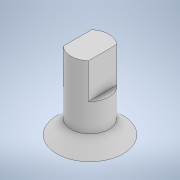
# Autodesk Inventor part: driven gear axle
Saved by Autodesk Inventor 2022 (Build 260153000, 153)
## iProperties
Created: 2021-11-11
Part Number: driven gear axle
Material: Generic
Document SubType Name: Modeling
Designer: a-dubs
Density: 1 g/cm^3
Appearance: Default
Author: a-dubs
Autodesk Inventor part; units mm, degrees
ref_plane "YZ Plane" through (0, 0, 0) normal (1, 0, 0) x (0, 1, 0)
ref_plane "XZ Plane" through (0, 0, 0) normal (0, 1, 0) x (-1, 0, 0)
ref_plane "XY Plane" through (0, 0, 0) normal (0, 0, 1) x (1, 0, 0)
sketch "Sketch1" plane through (0, 0, 0) normal (0, 1, 0) x (-1, 0, 0)
  line L0 (0, 0) -> (1.8, 0)
  line L1 (0, 0) -> (-1.8, 0)
  circle A0 centre (0, 0) radius 2.7
  line L2 (1.8, 0) -> (1.8, 2.0125)
  line L3 (1.8, 0) -> (1.8, -2.0125)
  line L4 (-1.8, 0) -> (-1.8, -2.0125)
  line L5 (-1.8, 0) -> (-1.8, 2.0125)
  circle A1 centre (0, 0) radius 4.7
  dimension "d0" = 1.8
  dimension "d1" = 1.8
  dimension "d2" = 5.4
  dimension "d7" = 9.4
  constraints: 12 end point, 4 point on circle, 2 centre point, 2 coincident, 2 horizontal, 2 point on line, 1 parallel, 1 vertical
  measures "d0" distance of L0.start L0.end
  measures "d1" distance of L0.start L1.end
  measures "d2" diameter of A0
  measures "d7" diameter of A1
extrude "Extrusion1" add sketch "Sketch1" along normal blind 4 contours L1 L5 A0 L2 L0 | L0 L3 A0 L4 L1 | L2 A0 L3 | L4 A0 L5
extrude "Extrusion2" add sketch "Sketch1" along normal blind 5 from surface at 4 contours L1 L5 A0 L2 L0 | L0 L3 A0 L4 L1
extrude "Extrusion3" add sketch "Sketch1" against normal blind 2 contours L1 L5 A0 L2 L0 | L0 L3 A0 L4 L1 | L2 A0 L3 | L4 A0 L5 | A1
chamfer "Chamfer1" distance 2 angle 45 1 edges at (4.7, 0, 0)
body "Solid1"
